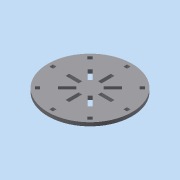
# Autodesk Inventor part: base
Saved by Autodesk Inventor 2015 (Build 190159000, 159)
## iProperties
Created: 2017-10-02
Part Number: base
Material: Generic
Document SubType Name: Modeling
Designer: macbook
Density: 1 g/cm^3
Appearance: Default
Author: macbook
Autodesk Inventor part; units mm, degrees
ref_plane "YZ Plane" through (0, 0, 0) normal (1, 0, 0) x (0, 1, 0)
ref_plane "XZ Plane" through (0, 0, 0) normal (0, 1, 0) x (-1, 0, 0)
ref_plane "XY Plane" through (0, 0, 0) normal (0, 0, 1) x (1, 0, 0)
sketch "Sketch1" plane through (0, 0, 0) normal (0, 0, 1) x (1, 0, 0)
  circle A0 centre (0, 0) radius 65
  dimension "d0" = 130
  constraints: 1 centre point, 1 coincident
  measures "d0" diameter of A0
extrude "Extrusion1" add sketch "Sketch1" along normal blind 5.5
sketch "Sketch4" plane through (0, 0, 5.5) normal (0, 0, 1) x (1, 0, 0)
  line L0 (15, -2.7) -> (15, 2.8)
  line L1 (8.6974, 12.6158) -> (22.8395, 26.7579)
  line L2 (22.8395, 26.7579) -> (26.7286, 22.8688)
  line L3 (26.7286, 22.8688) -> (12.5865, 8.7267)
  line L4 (-8.6267, 12.6865) -> (-12.5158, 8.7974)
  line L5 (-12.5158, 8.7974) -> (-26.6579, 22.9395)
  line L6 (-26.6579, 22.9395) -> (-22.7688, 26.8286)
  line L7 (-22.7688, 26.8286) -> (-8.6267, 12.6865)
  line L8 (2.8, 15.1) -> (-2.7, 15.1)
  line L9 (12.5865, 8.7267) -> (8.6974, 12.6158)
  line L10 (-2.7, 15.1) -> (-2.7, 35.1)
  line L11 (-2.7, 35.1) -> (2.8, 35.1)
  line L12 (2.8, 35.1) -> (2.8, 15.1)
  line L13 (-15, 2.9) -> (-15, -2.6)
  line L14 (-35, 2.9) -> (-15, 2.9)
  line L15 (-35, -2.6) -> (-35, 2.9)
  line L16 (-15, -2.6) -> (-35, -2.6)
  line L17 (-12.5865, -8.5267) -> (-8.6974, -12.4158)
  line L18 (-26.7286, -22.6688) -> (-12.5865, -8.5267)
  line L19 (-8.6974, -12.4158) -> (-22.8395, -26.5579)
  line L20 (-22.8395, -26.5579) -> (-26.7286, -22.6688)
  line L21 (15, 2.8) -> (35, 2.8)
  line L22 (35, 2.8) -> (35, -2.7)
  line L23 (35, -2.7) -> (15, -2.7)
  line L24 (-2.8, -14.9) -> (2.7, -14.9)
  line L25 (8.6267, -12.4865) -> (12.5158, -8.5974)
  line L26 (2.7, -14.9) -> (2.7, -34.9)
  line L27 (2.7, -34.9) -> (-2.8, -34.9)
  line L28 (22.7688, -26.6286) -> (8.6267, -12.4865)
  line L29 (12.5158, -8.5974) -> (26.6579, -22.7395)
  line L30 (26.6579, -22.7395) -> (22.7688, -26.6286)
  line L31 (-2.8, -34.9) -> (-2.8, -14.9)
  line L32 (24.2998, 0.05) -> (27.4417, 0.05)
  point P0 (0, 0)
  point P1 (0, 0)
  point P2 (0, 0)
  point P3 (0, 0.1)
  dimension "d21" = 20
  dimension "d22" = 5.5
  dimension "d23" = 360
  dimension "d24" = 2.75
  constraints: 66 end point, 2 horizontal, 2 parallel, 1 coincident, 1 perpendicular, 65 other
  measures "d21" distance of L23.start L23.end
  measures "d22" distance of L21.end L23.start
  measures "d24" distance between parallel lines of L21 L32
extrude "Extrusion4" cut sketch "Sketch4" against normal blind 10
sketch "Sketch5" plane through (0, 0, 5.5) normal (0, 0, 1) x (1, 0, 0)
  line L0 (54.5, 2.75) -> (60, 2.75)
  line L1 (60, 2.75) -> (60, -2.75)
  line L2 (60, -2.75) -> (54.5, -2.75)
  line L3 (54.5, -2.75) -> (54.5, 2.75)
  line L4 (36.5928, 40.4819) -> (40.4819, 44.371)
  line L5 (40.4819, 44.371) -> (44.371, 40.4819)
  line L6 (44.371, 40.4819) -> (40.4819, 36.5928)
  line L7 (40.4819, 36.5928) -> (36.5928, 40.4819)
  line L8 (-2.75, 54.5) -> (-2.75, 60)
  line L9 (-2.75, 60) -> (2.75, 60)
  line L10 (2.75, 60) -> (2.75, 54.5)
  line L11 (2.75, 54.5) -> (-2.75, 54.5)
  line L12 (-40.4819, 36.5928) -> (-44.371, 40.4819)
  line L13 (-44.371, 40.4819) -> (-40.4819, 44.371)
  line L14 (-40.4819, 44.371) -> (-36.5928, 40.4819)
  line L15 (-36.5928, 40.4819) -> (-40.4819, 36.5928)
  line L16 (-54.5, -2.75) -> (-60, -2.75)
  line L17 (-60, -2.75) -> (-60, 2.75)
  line L18 (-60, 2.75) -> (-54.5, 2.75)
  line L19 (-54.5, 2.75) -> (-54.5, -2.75)
  line L20 (-36.5928, -40.4819) -> (-40.4819, -44.371)
  line L21 (-40.4819, -44.371) -> (-44.371, -40.4819)
  line L22 (-44.371, -40.4819) -> (-40.4819, -36.5928)
  line L23 (-40.4819, -36.5928) -> (-36.5928, -40.4819)
  line L24 (2.75, -54.5) -> (2.75, -60)
  line L25 (2.75, -60) -> (-2.75, -60)
  line L26 (-2.75, -60) -> (-2.75, -54.5)
  line L27 (-2.75, -54.5) -> (2.75, -54.5)
  line L28 (40.4819, -36.5928) -> (44.371, -40.4819)
  line L29 (44.371, -40.4819) -> (40.4819, -44.371)
  line L30 (40.4819, -44.371) -> (36.5928, -40.4819)
  line L31 (36.5928, -40.4819) -> (40.4819, -36.5928)
  point P0 (0, 0)
  dimension "d30" = 5.5
  dimension "d31" = 5.5
  dimension "d34" = 360
  constraints: 64 end point, 2 parallel, 1 horizontal, 1 perpendicular, 65 other
  measures "d30" distance of L1.end L2.end
  measures "d31" distance of L0.end L1.end
extrude "Extrusion5" cut sketch "Sketch5" against normal blind 10
body "Solid1"
